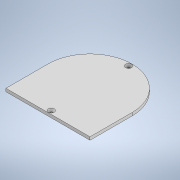
# Autodesk Inventor part: base-bottom-2
Saved by Autodesk Inventor 2021 (Build 250183000, 183)
## iProperties
Created: 2021-03-20
Part Number: base-bottom-2
Material: Generic
Document SubType Name: Modeling
Designer: Kayla
Density: 1 g/cm^3
Appearance: Default
Author: Kayla
Autodesk Inventor part; units mm, degrees
ref_plane "YZ Plane" through (0, 0, 0) normal (1, 0, 0) x (0, 1, 0)
ref_plane "XZ Plane" through (0, 0, 0) normal (0, 1, 0) x (-1, 0, 0)
ref_plane "XY Plane" through (0, 0, 0) normal (0, 0, 1) x (1, 0, 0)
sketch "Sketch1" plane through (0, 0, 0) normal (0, 1, 0) x (-1, 0, 0)
  line L0 (30.0636, 48.5262) -> (-81.1364, 48.5262)
  line L1 (-81.1364, 48.5262) -> (-81.1364, -7.0738)
  line L2 (-81.1364, -7.0738) -> (30.0636, -7.0738)
  line L3 (30.0636, -7.0738) -> (30.0636, 48.5262)
  arc A0 (-81.1364, -7.0738) -> (30.0636, -7.0738) centre (-25.5364, -7.0738) ccw
  point P0 (0, 0)
  dimension "d0" = 55.6
  dimension "d1" = 111.2
  dimension "d2" = 55.6
  constraints: 8 end point, 2 parallel, 2 point on circle, 1 centre point, 1 horizontal, 1 perpendicular
  measures "d0" distance of L2.end L0.start
  measures "d1" distance of L0.start L0.end
  measures "d2" radius of A0
extrude "Extrusion1" add sketch "Sketch1" along normal blind 4
sketch "Sketch2" plane through (0, 4, 0) normal (0, 1, 0) x (1, 0, 0)
  line L0 (-30.0636, 7.0738) -> (-30.0636, -48.5262) projected
  line L1 (-30.0636, -48.5262) -> (81.1364, -48.5262) projected
  point P0 (0, 0)
  point P1 (25.5364, -44.0432)
  dimension "d12" = 55.6
  dimension "d13" = 4.483
  measures "d12" distance from line of L0 point (25.536, -44.043)
  measures "d13" distance from line of L1 point (25.536, -44.043)
hole "Hole1" at (25.5364, 4, 44.0432) direction (0, -1, 0) diameter 3 depth 5 tip angle 118 countersink diameter 8 countersink angle 90
sketch "Sketch3" plane through (0, 4, 0) normal (0, 1, 0) x (1, 0, 0)
  line L0 (-30.0636, 7.0738) -> (-30.0636, -48.5262) projected
  arc A0 (81.1364, 7.0738) -> (-30.0636, 7.0738) centre (25.5364, 7.0738) ccw projected
  point P0 (0, 0)
  point P1 (25.5364, 58.1228)
  dimension "d21" = 55.6
  dimension "d22" = 51.049
  measures "d21" distance from line of L0 point (25.536, 58.123)
  measures "d22" distance of A0.centre point (25.536, 58.123)
hole "Hole2" at (25.5364, 4, -58.1228) direction (0, -1, 0) diameter 3 depth 5 tip angle 118 countersink diameter 8 countersink angle 90
body "Solid1"
